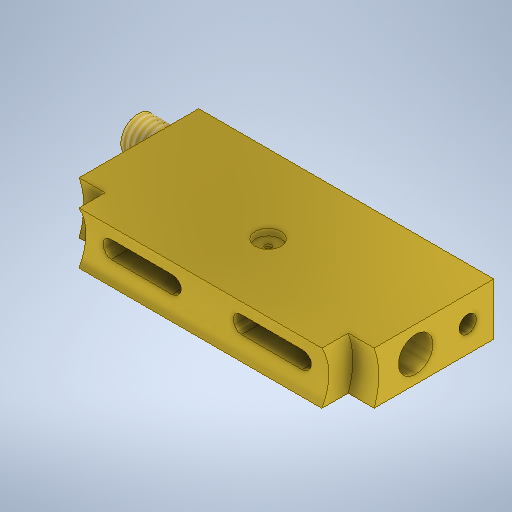
# Autodesk Inventor part: 152
Saved by Autodesk Inventor 2025.1 (Build 291241000, 241)
## iProperties
Created: 2024-08-03
Part Number: 152
Material: Gold
Document SubType Name: Modeling
Designer: ffogue
Density: 19.3 g/cm^3
Appearance: Metal 2400F Hot
Author: ffogue
Autodesk Inventor part; units mm, degrees
ref_plane "XZ Plane" through (0, 0, 0) normal (0, 1, 0) x (-1, 0, 0)
ref_plane "XY Plane" through (0, 0, 0) normal (0, 0, 1) x (1, 0, 0)
sketch "Sketch1" plane through (0, 0, 0) normal (0, 0, 1) x (1, 0, 0)
  line L0 (0, 0) -> (-28, 0)
  line L1 (-28, 0) -> (-28, 4.5)
  line L2 (-28, 4.5) -> (-34, 4.5)
  line L3 (-34, 4.5) -> (-34, 36)
  line L4 (-34, 36) -> (34, 36)
  line L5 (34, 36) -> (34, 4.5)
  line L6 (34, 4.5) -> (28, 4.5)
  line L7 (28, 4.5) -> (28, 0)
  line L8 (28, 0) -> (0, 0)
  line L9 (0, 0) -> (0, 8.4212) construction
  dimension "d0" = 28
  dimension "d1" = 28
  dimension "d2" = 68
  dimension "d3" = 36
  dimension "d4" = 4.5
  constraints: 20 end point, 6 perpendicular, 3 point on line, 1 collinear, 1 horizontal, 1 vertical, 1 other
  measures "d0" distance of L0.start L0.end
  measures "d1" distance of L7.end L0.start
  measures "d2" distance of L3.end L4.end
  measures "d3" distance between parallel lines of L8 L4
  measures "d4" distance between parallel lines of L0 L2
extrude "Extrusion1" add sketch "Sketch1" along normal mid plane 12
ref_plane "Work Plane3" through (-28, 0, 0) normal (1, 0, 0) x (0, 1, 0)
sketch "Sketch12" plane through (-28, 0, 0) normal (1, 0, 0) x (0, 1, 0)
  circle A0 centre (30, 0) radius 4
  line L0 (36, -6) -> (36, 6) projected
  point P0 (0, 0)
  point P1 (36, 0)
  dimension "d61" = 8
  dimension "d62" = 6
  constraints: 1 centre point, 1 horizontal alignment, 1 midpoint
  measures "d61" diameter of A0
  measures "d62" distance from line of L0 A0.centre
extrude "Extrusion5" add sketch "Sketch12" against normal blind 14
sketch "Sketch2" plane through (0, 0, 6) normal (0, 0, 1) x (1, 0, 0)
  line L0 (34, 36) -> (-34, 36) projected
  line L1 (-28, 0) -> (28, 0) projected
  point P0 (0, 0)
  point P1 (0, 18)
  point P2 (0, 36)
  point P3 (0, 0)
  dimension "d7" = 18
  constraints: 2 midpoint, 1 vertical alignment
  measures "d7" distance of point (0, 36) point (0, 18)
hole "Hole1" at (0, 18, 6) direction (0, 0, -1) diameter 1.5 depth 12 counterbore diameter 6 counterbore depth 1.5
sketch "Sketch13" plane through (-42, 30, 0) normal (-1, 0, 0) x (0, 0, 1)
  circle A0 centre (0, 0) radius 4 projected
  point P0 (0, -30)
  constraints: 1 coincident
hole "Hole6" at (-42, 30, 0) direction (1, 0, 0) diameter 4 depth 76 counterbore diameter 5 counterbore depth 9
sketch "Sketch4" plane through (-34, 4.5, 6) normal (-1, 0, 0) x (0, 0, 1)
  circle A0 centre (-6, 25.5) radius 2.067 projected
  point P0 (-6, -4.5)
  point P1 (-6, 13.5)
  dimension "d23" = 12
  constraints: 1 vertical alignment
  measures "d23" distance of point (-6, 13.5) A0.centre
hole "Hole3" at (-34, 18, 0) direction (1, 0, 0) diameter 8 depth 68
sketch "Sketch5" plane through (-28, 0, 6) normal (0, -1, 0) x (1, 0, 0)
  line L0 (-6, -12) -> (-6, 0) projected
  line L1 (62, -12) -> (62, 0) projected
  point P0 (28, -6)
  point P1 (6, -6)
  point P2 (50, -6)
  point P3 (-6, -6)
  dimension "d31" = 12
  dimension "d32" = 12
  constraints: 2 horizontal alignment, 1 midpoint
  measures "d31" distance of point (-6, -6) point (6, -6)
  measures "d32" distance from line of L1 point (50, -6)
hole "Hole4" at (-22, 0, 0) at (22, 0, 0) direction (0, 1, 0) diameter 4 depth 36
sketch "Sketch6" plane through (-28, 0, 6) normal (0, -1, 0) x (1, 0, 0)
  point P0 (28, -6)
  point P1 (20, -6)
  point P2 (36, -6)
  dimension "d40" = 8
  dimension "d41" = 8
  constraints: 2 horizontal alignment
  measures "d40" distance of point (28, -6) point (20, -6)
  measures "d41" distance of point (28, -6) point (36, -6)
hole "Hole5" at (-8, 0, 0) at (8, 0, 0) direction (0, 1, 0) diameter 4 depth 14.5
sketch "Sketch10" plane through (-28, 0, 6) normal (0, -1, 0) x (1, 0, 0)
  circle A0 centre (6, -6) radius 2 projected
  circle A1 centre (20, -6) radius 2 projected
  line L0 (6, -4) -> (20.1253, -4)
  line L1 (20, -8) -> (6, -8)
  point P0 (28, -6)
  point P1 (20, -4)
  constraints: 4 end point, 3 horizontal, 4 other
extrude "Extrusion4" cut sketch "Sketch10" against normal blind 8 contours A0 L0 A1 L1
mirror "Mirror2" about plane through (0, 0, 0) normal (1, 0, 0) of "Extrusion4"
sketch "Sketch7" plane through (-34, 4.5, 6) normal (-1, 0, 0) x (0, 0, 1)
  arc A0 (0, -2.1077) -> (-12, -2.1077) centre (-6, -12.5) ccw
  line L0 (-12, -4.5) -> (0, -4.5) projected
  line L1 (0, 0) -> (0, -4.5) projected
  line L2 (-12, 0) -> (0, 0) projected
  line L3 (-12, -4.5) -> (-12, 0) projected
  circle A1 centre (-6, 13.5) radius 4 projected
  point P0 (-6, -4.5)
  dimension "d49" = 24
  dimension "d50" = 26
  constraints: 2 point on circle, 2 point on line, 1 centre point, 1 vertical alignment
  measures "d49" diameter of A0
  measures "d50" distance of A0.centre A1.centre
extrude "Extrusion2" cut sketch "Sketch7" against normal up to surface (68 mm away) contours L1 L0 L3 A0
sketch "Sketch8" plane through (-34, 4.5, 6) normal (-1, 0, 0) x (0, 0, 1)
  arc A0 (0, 3.9393) -> (-12, 3.9393) centre (-6, -12.5) ccw
  arc A1 (0, -2.1077) -> (-12, -2.1077) centre (-6, -12.5) ccw projected
  line L0 (0, 31.5) -> (0, 0) projected
  line L1 (-12, 0) -> (-12, 31.5) projected
  line L2 (-12, 0) -> (0, 0) projected
  point P0 (-6, -4.5)
  point P1 (-6, 0)
  dimension "d53" = 35
  constraints: 2 point on circle, 2 point on line, 1 centre point, 1 concentric
  measures "d53" diameter of A0
extrude "Extrusion3" cut sketch "Sketch8" against normal up to surface (6 mm away)
mirror "Mirror1" about plane through (0, 0, 0) normal (1, 0, 0) of "Extrusion3"
thread "Thread1" size "M8x1.25" class "6g" standard "ISO Metric profile" full length
equation "\"d41\" = d40"
body "Solid1"
